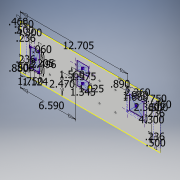
# Autodesk Inventor part: PDU_chassis_back
Saved by Autodesk Inventor 2017 (Build 210142000, 142)
## iProperties
Created: 2017-02-14
Part Number: PDU_chassis_back
Material: Generic
Document SubType Name: Modeling
Designer: Zara
Density: 1 g/cm^3
Appearance: Default
Author: Zara
Autodesk Inventor part; units mm, degrees
ref_plane "YZ Plane" through (0, 0, 0) normal (1, 0, 0) x (0, 1, 0)
ref_plane "XZ Plane" through (0, 0, 0) normal (0, 1, 0) x (-1, 0, 0)
ref_plane "XY Plane" through (0, 0, 0) normal (0, 0, 1) x (1, 0, 0)
sketch "Sketch1" plane through (0, 0, 0) normal (0, 0, 1) x (1, 0, 0)
  line L0 (-209.423, -66.294) -> (209.423, -66.294)
  line L1 (209.423, -66.294) -> (209.423, 66.294)
  line L2 (209.423, 66.294) -> (-209.423, 66.294)
  line L3 (-209.423, 66.294) -> (-209.423, -66.294)
  line L4 (-209.423, -66.294) -> (209.423, 66.294) construction
  line L5 (209.423, -66.294) -> (-209.423, 66.294) construction
  point P0 (0, 0)
  dimension "d0" = 418.846
  dimension "d1" = 132.588
  constraints: 12 end point, 2 midpoint, 2 parallel, 1 horizontal, 1 perpendicular
  measures "d0" distance of L1.end L2.end
  measures "d1" distance of L0.end L1.end
extrude "PDU back" add sketch "Sketch1" along normal blind 1.651
sketch "pwr entry" plane through (0, 0, 1.651) normal (0, 0, 1) x (1, 0, 0)
  line L0 (-177.7238, -40.259) -> (-152.2222, -40.259)
  line L1 (-150.6982, -38.735) -> (-150.6982, 14.224)
  line L2 (-152.2222, 15.748) -> (-177.7238, 15.748)
  line L3 (-179.2478, 14.224) -> (-179.2478, -38.735)
  line L4 (-179.2478, -40.259) -> (-150.6982, 15.748) construction
  line L5 (-150.6982, -40.259) -> (-179.2478, 15.748) construction
  line L6 (-164.973, 19.4437) -> (-164.973, -43.9547) construction
  line L7 (-209.423, 66.294) -> (-209.423, -66.294) projected
  line L8 (-209.423, -66.294) -> (209.423, -66.294) projected
  arc A0 (-150.6982, 14.224) -> (-152.2222, 15.748) centre (-152.2222, 14.224) ccw
  arc A1 (-177.7238, 15.748) -> (-179.2478, 14.224) centre (-177.7238, 14.224) ccw
  arc A2 (-179.2478, -38.735) -> (-177.7238, -40.259) centre (-177.7238, -38.735) ccw
  arc A3 (-152.2222, -40.259) -> (-150.6982, -38.735) centre (-152.2222, -38.735) ccw
  point P0 (0, 0)
  point P1 (-164.973, -12.2555)
  point P2 (-164.973, -12.2555)
  dimension "d4" = 56.007
  dimension "d5" = 28.5496
  dimension "d6" = 63.3984
  dimension "d7" = 44.45
  dimension "d8" = 22.3393
  dimension "d9" = 1.524
  constraints: 14 end point, 8 point on circle, 8 point on line, 8 tangent, 4 centre point, 4 midpoint, 3 equal radius, 2 coincident, 2 parallel, 1 horizontal, 1 perpendicular, 1 vertical
  measures "d4" distance of L5.start L4.end
  measures "d5" distance of L4.start L5.start
  measures "d6" distance of L6.end L6.start
  measures "d7" distance from line of L7 L6.end
  measures "d8" distance from line of point (-164.973, -43.955) L8
  measures "d9" radius of A0
extrude "pwr entry cutout" cut sketch "pwr entry" against normal through all
hole "pwr entry holes" at (-164.973, 19.4437, 1.651) at (-164.973, -43.9547, 1.651) direction (0, 0, -1) diameter 3.4544 end through all
sketch "IEC outlet" plane through (0, 0, 1.651) normal (0, 0, 1) x (1, 0, 0)
  line L0 (-39.116, -16.5735) -> (-4.953, -16.5735)
  line L1 (-4.953, -16.5735) -> (-4.953, 9.4615)
  line L2 (-4.953, 9.4615) -> (-39.116, 9.4615)
  line L3 (-39.116, 9.4615) -> (-39.116, -16.5735)
  line L4 (-39.116, -16.5735) -> (-4.953, 9.4615) construction
  line L5 (-4.953, -16.5735) -> (-39.116, 9.4615) construction
  line L6 (-42.037, -3.556) -> (-2.032, -3.556) construction
  line L7 (-209.423, 66.294) -> (-209.423, -66.294) projected
  line L8 (-209.423, -66.294) -> (209.423, -66.294) projected
  line L9 (-39.116, 23.0505) -> (-4.953, 23.0505)
  line L10 (-4.953, 23.0505) -> (-4.953, 49.0855)
  line L11 (-4.953, 49.0855) -> (-39.116, 49.0855)
  line L12 (-39.116, 49.0855) -> (-39.116, 23.0505)
  line L13 (-39.116, 23.0505) -> (-4.953, 49.0855) construction
  line L14 (-4.953, 23.0505) -> (-39.116, 49.0855) construction
  line L15 (-42.037, 36.068) -> (-2.032, 36.068) construction
  point P0 (-22.0345, -3.556)
  point P1 (-22.0345, -3.556)
  point P2 (-22.0345, 36.068)
  point P3 (-22.0345, 36.068)
  dimension "d19" = 26.035
  dimension "d20" = 34.163
  dimension "d22" = 40.005
  dimension "d23" = 167.386
  dimension "d24" = 62.738
  dimension "d129" = 39.624
  constraints: 28 end point, 6 midpoint, 4 coincident, 2 horizontal, 2 parallel, 1 collinear, 1 perpendicular, 1 vertical, 16 other
  measures "d19" distance of L0.end L1.end
  measures "d20" distance of L0.start L0.end
  measures "d22" distance of L6.end point (-42.037, -3.556)
  measures "d23" distance from line of L7 L6.start
  measures "d24" distance from line of L6.start L8
  measures "d129" distance of L0.start L9.start
hole "IEC holes" at (-2.032, -3.556, 1.651) at (-42.037, -3.556, 1.651) at (-2.032, 36.068, 1.651) at (-42.037, 36.068, 1.651) direction (0, 0, -1) diameter 3.4544 end through all
sketch "airflow" plane through (0, 0, 1.651) normal (0, 0, 1) x (1, 0, 0)
  line L0 (-209.423, 66.294) -> (-209.423, -66.294) projected
  line L1 (-209.423, -66.294) -> (209.423, -66.294) projected
  line L2 (108.331, -11.303) -> (168.275, -11.303) construction
  line L3 (168.275, -11.303) -> (168.275, 48.641) construction
  line L4 (168.275, 48.641) -> (108.331, 48.641) construction
  line L5 (108.331, 48.641) -> (108.331, -11.303) construction
  line L6 (108.331, -11.303) -> (168.275, 48.641) construction
  line L7 (168.275, -11.303) -> (108.331, 48.641) construction
  line L8 (113.284, -6.35) -> (163.322, -6.35) construction
  line L9 (163.322, -6.35) -> (163.322, 43.688) construction
  line L10 (163.322, 43.688) -> (113.284, 43.688) construction
  line L11 (113.284, 43.688) -> (113.284, -6.35) construction
  line L12 (113.284, -6.35) -> (163.322, 43.688) construction
  line L13 (163.322, -6.35) -> (113.284, 43.688) construction
  line L14 (117.221, -2.413) -> (159.385, -2.413)
  line L15 (159.385, -2.413) -> (159.385, 39.751)
  line L16 (159.385, 39.751) -> (117.221, 39.751)
  line L17 (117.221, 39.751) -> (117.221, -2.413)
  line L18 (117.221, -2.413) -> (159.385, 39.751) construction
  line L19 (159.385, -2.413) -> (117.221, 39.751) construction
  line L20 (209.423, 66.294) -> (-209.423, 66.294) projected
  point P0 (0, 0)
  point P1 (138.303, 18.669)
  point P2 (138.303, 18.669)
  dimension "d76" = 59.944
  dimension "d77" = 59.944
  dimension "d78" = 50.038
  dimension "d79" = 42.164
  dimension "d123" = 22.606
  dimension "d153" = 322.707
  constraints: 36 end point, 8 midpoint, 6 parallel, 4 coincident, 3 horizontal, 3 perpendicular, 2 point on line
  measures "d76" distance of L3.end L4.end
  measures "d77" distance of L2.end L3.end
  measures "d78" distance of L9.end L10.end
  measures "d79" distance of L15.end L16.end
  measures "d123" distance from line of L20 point (113.284, 43.688)
  measures "d153" distance from line of L0 point (113.284, 43.688)
sketch "relay holes" plane through (0, 0, 0) normal (0, 0, -1) x (-1, 0, 0)
  circle A0 centre (2.032, -3.556) radius 1.7272 construction
  line L0 (84.9503, 23.1654) -> (84.9503, -54.0444) construction
  line L1 (-209.423, 66.294) -> (209.423, 66.294) projected
  line L2 (5.08, 36.068) -> (5.08, -3.9037) construction
  line L3 (150.6982, 14.224) -> (150.6982, -38.735) projected
  line L4 (72.4662, -29.21) -> (120.2182, -29.21) construction
  point P0 (-28.448, -29.21)
  point P1 (-28.448, 29.21)
  point P2 (-76.2, 29.21)
  point P3 (-76.2, -29.21)
  point P4 (-25.4, -29.21)
  point P5 (2.032, 36.068)
  dimension "d138" = 47.752
  dimension "d139" = 37.084
  dimension "d143" = 58.42
  dimension "d148" = 47.752
  dimension "d149" = 95.504
  dimension "d150" = 30.48
  dimension "d175" = 30.48
  dimension "d176" = 47.752
  dimension "d177" = 30.48
  constraints: 6 end point, 1 horizontal, 1 vertical
  measures "d138" distance of point (-76.2, 29.21) point (-28.448, 29.21)
  measures "d139" distance from line of point (-28.448, 29.21) L1
  measures "d143" distance of point (-76.2, 29.21) point (-76.2, -29.21)
  measures "d148" distance of L4.end L4.start
  measures "d149" distance between parallel lines of L1 L4
  measures "d150" distance from line of L3 L4.end
  measures "d175" horizontal distance of point (2.032, -3.556) point (-28.448, -29.21)
  measures "d176" distance of point (-28.448, -29.21) point (-76.2, -29.21)
  measures "d177" horizontal distance of point (2.032, 36.068) point (-28.448, 29.21)
hole "Hole5" at (163.322, 43.688, 1.651) at (113.284, 43.688, 1.651) at (113.284, -6.35, 1.651) at (163.322, -6.35, 1.651) direction (0, 0, -1) diameter 4.4958 end through all clearance for "Flat Head Machine Screw (82)" size "#8" standard "Ansi Unified Screw Threads"
extrude "Extrusion6" cut sketch "airflow" against normal blind 25.4
sketch "bracket" plane through (0, 0, 1.651) normal (0, 0, 1) x (1, 0, 0)
  line L0 (209.423, -66.294) -> (209.423, 66.294) construction
  line L1 (209.423, 54.61) -> (190.373, 54.61) construction
  line L2 (190.373, 54.61) -> (190.373, -54.61) construction
  line L3 (190.373, -54.61) -> (209.423, -54.61) construction
  line L4 (209.423, -54.61) -> (209.423, 54.61) construction
  line L5 (209.423, 66.294) -> (-209.423, 66.294) construction
  line L6 (-209.423, 66.294) -> (-209.423, -66.294) construction
  line L7 (-209.423, 54.61) -> (-190.373, 54.61) construction
  line L8 (-190.373, 54.61) -> (-190.373, -54.61) construction
  line L9 (-190.373, -54.61) -> (-209.423, -54.61) construction
  line L10 (-209.423, -54.61) -> (-209.423, 54.61) construction
  point P0 (0, 0)
  point P1 (196.3674, 41.91)
  point P2 (196.3674, -41.91)
  point P3 (-196.3674, -41.91)
  point P4 (-196.3674, 41.91)
  dimension "d94" = 19.05
  dimension "d95" = 109.22
  dimension "d96" = 11.684
  dimension "d103" = 19.05
  dimension "d104" = 109.22
  dimension "d105" = 11.684
  dimension "d121" = 12.7
  dimension "d122" = 5.9944
  dimension "d161" = 12.7
  dimension "d162" = 12.7
  dimension "d163" = 5.9944
  dimension "d164" = 5.9944
  dimension "d165" = 12.7
  dimension "d166" = 5.9944
  constraints: 16 end point, 4 parallel, 2 horizontal, 2 perpendicular, 2 point on line
  measures "d94" distance of L1.start L1.end
  measures "d95" distance of L1.end L2.end
  measures "d96" distance between parallel lines of L5 L1
  measures "d103" distance of L7.start L7.end
  measures "d104" distance of L7.end L8.end
  measures "d105" distance between parallel lines of L5 L7
  measures "d121" distance from line of L1 point (196.367, 41.91)
  measures "d122" distance from line of L2 point (196.367, 41.91)
  measures "d161" distance from line of point (-196.367, 41.91) L7
  measures "d162" distance from line of point (-196.367, -41.91) L9
  measures "d163" distance from line of L8 point (-196.367, -41.91)
  measures "d164" distance from line of point (-196.367, 41.91) L8
  measures "d165" distance from line of point (196.367, -41.91) L3
  measures "d166" distance from line of L2 point (196.367, -41.91)
hole "bracket holes" at (-196.3674, 41.91, 1.651) at (-196.3674, -41.91, 1.651) at (196.3674, 41.91, 1.651) at (196.3674, -41.91, 1.651) direction (0, 0, -1) diameter 4.2926 end through all clearance for "Countersunk Flat Head Screw ISO 2009/7046" size "M4" standard "ISO"
extrude "Extrusion7" cut sketch "IEC outlet" against normal through all
fillet "Fillet3" radius 4.9784 8 edges at (-39.116, 49.0855, 0.8255) (-39.116, 23.0505, 0.8255) (-4.953, 23.0505, 0.8255) (-4.953, 49.0855, 0.8255) (-4.953, 9.4615, 0.8255) (-39.116, 9.4615, 0.8255) (-39.116, -16.5735, 0.8255) (-4.953, -16.5735, 0.8255)
hole "Hole8" at (28.448, 29.21, 0) at (76.2, 29.21, 0) at (76.2, -29.21, 0) at (28.448, -29.21, 0) at (-120.2182, -29.21, 0) at (-72.4662, -29.21, 0) direction (0, 0, 1) diameter 4.4958 end through all clearance for "Flat Head Machine Screw (82)" size "#8" standard "Ansi Unified Screw Threads"
body "Solid1"
